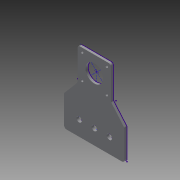
# Autodesk Inventor part: y_motor_mount
Saved by Autodesk Inventor 2013 (Build 170138000, 138)
## iProperties
Created: 2013-09-20
Part Number: y_motor_mount
Material: Generic
Document SubType Name: Modeling
Designer: Ian
Density: 1 g/cm^3
Mass: 16.7632 g
Surface Area: 121.435 cm^2
Volume: 16.7632 cm^3
Author: Ian
Autodesk Inventor part; units mm, degrees
ref_plane "YZ Plane" through (0, 0, 0) normal (1, 0, 0) x (0, 1, 0)
ref_plane "XZ Plane" through (0, 0, 0) normal (0, 1, 0) x (-1, 0, 0)
ref_plane "XY Plane" through (0, 0, 0) normal (0, 0, 1) x (1, 0, 0)
sketch "Sketch1" plane through (0, 0, 0) normal (0, 0, 1) x (1, 0, 0)
  line L0 (0, 0) -> (0, 40.5892) construction
  line L1 (0, 0) -> (0, -19.05) construction
  circle A0 centre (0, 40.5892) radius 11
  line L2 (-15.5, 25.0892) -> (15.5, 25.0892) construction
  line L3 (15.5, 25.0892) -> (15.5, 56.0892) construction
  line L4 (15.5, 56.0892) -> (-15.5, 56.0892) construction
  line L5 (-15.5, 56.0892) -> (-15.5, 25.0892) construction
  line L6 (-15.5, 25.0892) -> (15.5, 56.0892) construction
  line L7 (15.5, 25.0892) -> (-15.5, 56.0892) construction
  line L8 (-21, 20.0892) -> (21, 20.0892) construction
  line L9 (21, 21.2575) -> (21, 57.9142)
  line L10 (17.825, 61.0892) -> (-17.825, 61.0892)
  line L11 (-21, 57.9142) -> (-21, 21.2575)
  line L12 (-21, 20.0892) -> (21, 61.0892) construction
  line L13 (21, 20.0892) -> (-21, 61.0892) construction
  line L14 (0, -19.05) -> (0, -38.1) construction
  line L15 (19.05, -19.05) -> (38.1, -19.05) construction
  line L16 (-19.05, -19.05) -> (-38.1, -19.05) construction
  line L17 (-34.925, -38.1) -> (34.925, -38.1)
  line L18 (38.1, -34.925) -> (38.1, -1.1683)
  line L19 (38.1, 0) -> (-38.1, 0) construction
  line L20 (-38.1, -1.1683) -> (-38.1, -34.925)
  line L21 (-21.7573, 19.1995) -> (-37.3427, 0.8897)
  line L22 (21.7573, 19.1995) -> (37.3427, 0.8897)
  arc A1 (-17.825, 61.0892) -> (-21, 57.9142) centre (-17.825, 57.9142) ccw
  arc A2 (-21.7573, 19.1995) -> (-21, 21.2575) centre (-24.175, 21.2575) ccw
  arc A3 (21, 21.2575) -> (21.7573, 19.1995) centre (24.175, 21.2575) ccw
  arc A4 (38.1, -1.1683) -> (37.3427, 0.8897) centre (34.925, -1.1683) ccw
  arc A5 (34.925, -38.1) -> (38.1, -34.925) centre (34.925, -34.925) ccw
  arc A6 (-38.1, -34.925) -> (-34.925, -38.1) centre (-34.925, -34.925) ccw
  arc A7 (-37.3427, 0.8897) -> (-38.1, -1.1683) centre (-34.925, -1.1683) ccw
  arc A8 (21, 57.9142) -> (17.825, 61.0892) centre (17.825, 57.9142) ccw
  point P0 (-38.1, -38.1)
  point P1 (38.1, -38.1)
  dimension "d0" = 40.5892
  dimension "d1" = 19.05
  dimension "d2" = 22
  dimension "d3" = 31
  dimension "d4" = 31
  dimension "d5" = 42
  dimension "d6" = 41
  dimension "d10" = 19.05
  dimension "d11" = 19.05
  dimension "d12" = 19.05
  dimension "d13" = 19.05
  dimension "d14" = 19.05
  dimension "d15" = 19.05
  dimension "d16" = 19.05
  dimension "d17" = 76.2
  dimension "d18" = 19.05
  dimension "d19" = 19.05
  dimension "d20" = 38.1
  dimension "d22" = 38.1
  dimension "d23" = 3.175
  dimension "d24" = 3.175
  dimension "d25" = 3.175
  constraints: 46 end point, 16 point on circle, 16 point on line, 16 tangent, 9 centre point, 7 coincident, 6 parallel, 5 equal radius, 4 midpoint, 4 perpendicular, 2 collinear, 2 horizontal, 1 vertical
  measures "d0" distance of L0.start L0.end
  measures "d1" distance of L0.start L1.end
  measures "d2" diameter of A0
  measures "d3" distance of L4.end L3.end
  measures "d4" distance of L3.end L2.end
  measures "d5" distance of L13.end L12.end
  measures "d6" distance of L12.end L8.end
  measures "d10" distance of L1.end L16.start
  measures "d11" distance of L1.end L15.start
  measures "d12" horizontal distance of L15.start L0.start
  measures "d13" horizontal distance of L16.start L0.start
  measures "d14" distance of L14.start L14.end
  measures "d15" distance of L15.start L15.end
  measures "d16" distance of L16.start L16.end
  measures "d17" distance of L19.start L19.end
  measures "d18" distance between parallel lines of L19 L15
  measures "d19" distance between parallel lines of L17 L15
  measures "d20" distance of point (-38.1, -38.1) L19.end
  measures "d22" distance of L14.end point (38.1, -38.1)
  measures "d23" radius of A1
  measures "d24" radius of A2
  measures "d25" radius of A8
extrude "Extrusion1" add sketch "Sketch1" along normal blind 3.175
hole "Hole1" at (0, -19.05, 0) at (0, 40.5892, 0) at (19.05, -19.05, 0) at (-19.05, -19.05, 0) direction (0, 0, 1) diameter 6.7564 end through all clearance for "Flat Head Machine Screw (82)" size "1/4" standard "Ansi Unified Screw Threads"
hole "Hole2" at (-15.5, 56.0892, 0) at (-15.5, 25.0892, 0) at (15.5, 25.0892, 0) at (15.5, 56.0892, 0) direction (0, 0, 1) diameter 3.4036 end through all clearance for "Flat Head Machine Screw" size "M3" standard "Ansi Metric M Profile"
body "Solid1"
